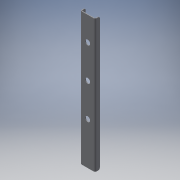
# Autodesk Inventor part: Soporte vertical
Saved by Autodesk Inventor 2016 (Build 200138000, 138)
## iProperties
Created: 2015-11-10
Part Number: Soporte vertical
Material: Generic
Document SubType Name: Sheet Metal
Designer: serge
Density: 1 g/cm^3
Sheet Metal Rule: Default
Appearance: Valor por defecto
Author: serge
Autodesk Inventor part; units mm, degrees
ref_plane "YZ Plane" through (0, 0, 0) normal (1, 0, 0) x (0, 1, 0)
ref_plane "XZ Plane" through (0, 0, 0) normal (0, 1, 0) x (-1, 0, 0)
ref_plane "XY Plane" through (0, 0, 0) normal (0, 0, 1) x (1, 0, 0)
sketch "Sketch1" plane through (0, 0, 0) normal (0, 0, 1) x (1, 0, 0)
  line L0 (-8.496, 0) -> (-8.496, 15)
  line L1 (-8.496, 0) -> (41.504, 0)
  line L2 (41.504, 0) -> (41.504, 15)
  point P0 (0, 0)
  dimension "d0" = 15
  dimension "d1" = 50
  dimension "d2" = 15
  measures "d0" distance of L0.start L0.end
  measures "d1" distance of L0.start L1.end
  measures "d2" distance of L1.end L2.end
contour flange "Contour Flange1" sketch "Sketch1" thickness 3 bend radius 3 width 498.475 along (0, 0, 1) mid plane no both sides no wall seen from (-8.496, 7.5, 0) lies toward (-1, 0, 0) curves L0 L1 L2
bend "Bend1"
corner "Corner1"
sketch "Sketch2" plane through (-5.496, -3, 498.475) normal (0, -1, 0) x (1, 0, 0)
  line L0 (44, 0) -> (44, -498.475) projected
  line L1 (0, 0) -> (44, 0) projected
  line L2 (0, -498.475) -> (44, -498.475) projected
  line L3 (22, 0) -> (22, -90)
  circle A0 centre (22, -90) radius 9.525
  point P0 (5.496, -498.475)
  dimension "d13" = 90
  dimension "diametro1" = 19.05
  dimension "d15" = 22
  constraints: 2 end point, 1 centre point, 1 coincident, 1 midpoint, 1 perpendicular
  measures "d13" distance of L3.start L3.end
  measures "diametro1" diameter of A0
  measures "d15" distance between parallel lines of L0 L3
extrude "Extrusion1" cut sketch "Sketch2" against normal blind 10
pattern_linear "Rectangular Pattern1" count 3 spacing 124.6188 along (0, 0, -1) of "Extrusion1"
fillet "Corner Round1" radius 6 4 edges at (43.004, 15, 0) (-9.996, 15, 0) (43.004, 15, 498.475) (-9.996, 15, 498.475)
equation "\"Distanciamiento\" = d_a2"
equation "\"d3\" = BendReliefWidth"
equation "\"d4\" = BendReliefDepth"
equation "\"d5\" = MinimumRemnant"
equation "\"d6\" = BendRadius"
equation "\"d8\" = BendRadius"
equation "\"d10\" = CornerReliefSize"
equation "\"d11\" = GapSize"
equation "\"d12\" = JacobiRadiusSize"
equation "\"Lon_ve\" = lon_ve2"
equation "\"BendRadius\" = Thickness"
equation "\"BendReliefWidth\" = Thickness"
equation "\"BendReliefDepth\" = 0.5 * Thickness"
equation "\"CornerReliefSize\" = 4 * Thickness"
equation "\"MinimumRemnant\" = 2 * Thickness"
equation "\"TransitionRadius\" = BendRadius"
equation "\"JacobiRadiusSize\" = Thickness"
equation "\"GapSize\" = Thickness"
equation "\"lon_ve2\" = 498.475"
equation "\"t_a2\" = 124.61875"
equation "\"d_a2\" = 124.61875"
equation "\"PE_N\" = 101.6"
equation "\"PE_S\" = 101.6"
equation "\"PE_EO\" = 101.6"
equation "\"T_E\" = 101.6"
equation "\"lon_ve\" = 512.5"
equation "\"n_a\" = 3"
equation "\"t_a\" = 19.05"
equation "\"d_a\" = 128.125"
equation "\"lon_ho\" = 749"
equation "\"d_bor\" = 59.92"
equation "\"lon_gui\" = 187.25"
equation "\"esp_gui\" = 461.25"
equation "\"n_a2\" = 3"
equation "\"lon_ho2\" = 933.45"
equation "\"d_bor2\" = 74.676"
equation "\"lon_gui2\" = 233.3625"
equation "\"esp_gui2\" = 448.6275"
equation "\"UE_L\" = 3435"
equation "\"UE_A\" = 1025"
equation "\"UE_AN\" = 749"
equation "\"UC_L\" = 1314.45"
equation "\"UC_A\" = 996.95"
equation "\"UC_AN\" = 933.45"
equation "\"A_ET\" = 35"
equation "\"SEP_NS\" = 0"
equation "\"DSEG\" = 0"
equation "\"AEGEP_NS\" = 0"
equation "\"DNS\" = 749"
equation "\"Thickness\" = 3"
body "Solid1"
